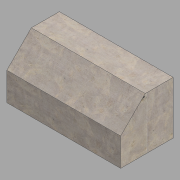
# Autodesk Inventor part: Full
Saved by Autodesk Inventor 2022.2 (Build 262287000, 287)
## iProperties
Created: 2021-12-31
Part Number: Full
Material: Limestone
Document SubType Name: Modeling
Designer: awelt
Density: 2.6 g/cm^3
Appearance: Kasota Gray
Mass: 42712.9 g
Surface Area: 4253.18 cm^2
Volume: 16428 cm^3
Author: awelt
Autodesk Inventor part; units mm, degrees
ref_plane "YZ Plane" through (0, 0, 0) normal (1, 0, 0) x (0, 1, 0)
ref_plane "XZ Plane" through (0, 0, 0) normal (0, 1, 0) x (-1, 0, 0)
ref_plane "XY Plane" through (0, 0, 0) normal (0, 0, 1) x (1, 0, 0)
sketch "Sketch1" plane through (0, 0, 0) normal (1, 0, 0) x (0, 1, 0)
  line L0 (0, 0) -> (190.5, 0)
  line L1 (0, 0) -> (0, 190.5)
  line L2 (190.5, 0) -> (190.5, 101.6)
  line L3 (0, 190.5) -> (101.6, 190.5)
  line L4 (101.6, 190.5) -> (190.5, 101.6)
  dimension "d0" = 190.5
  dimension "d1" = 190.5
  dimension "d2" = 101.6
  dimension "d3" = 101.6
  dimension "d4" = 88.9
  dimension "d5" = 88.9
  constraints: 10 end point, 2 horizontal, 2 vertical
  measures "d0" distance of L0.start L0.end
  measures "d1" distance of L0.start L1.end
  measures "d2" distance of L0.end L2.end
  measures "d3" distance of L1.end L3.end
  measures "d4" horizontal distance of L3.end L2.end
  measures "d5" horizontal distance of L3.end L2.end
extrude "Extrusion1" add sketch "Sketch1" along normal blind 412.75
body "Solid1"
